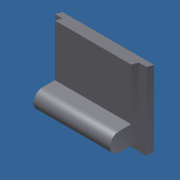
# Autodesk Inventor part: TETO DA CABINE(15)
Saved by Autodesk Inventor 2012 SP1 (Build 160190100, 190)
## iProperties
Created: 2012-07-23
Part Number: TETO DA CABINE(15)
Material: Carbon Steel
Document SubType Name: Modeling
Designer: bruno.silveira
Mass: 587.039 g
Surface Area: 115.824 cm^2
Volume: 74.592 cm^3
Density: 7.87 g/cm^3
Author: bruno.silveira
Autodesk Inventor part; units mm, degrees
ref_plane "YZ Plane" through (0, 0, 0) normal (1, 0, 0) x (0, 1, 0)
ref_plane "XZ Plane" through (0, 0, 0) normal (0, 1, 0) x (-1, 0, 0)
ref_plane "XY Plane" through (0, 0, 0) normal (0, 0, 1) x (1, 0, 0)
sketch "Sketch1" plane through (0, 0, 0) normal (0, 0, 1) x (1, 0, 0)
  line L0 (0, 0) -> (60, 0)
  line L1 (60, 0) -> (60, 24)
  line L2 (60, 24) -> (0, 24)
  line L3 (0, 24) -> (0, 0)
  dimension "d0" = 60
  dimension "d1" = 24
  constraints: 8 end point, 2 parallel, 1 horizontal, 1 perpendicular
  measures "d0" distance of L0.start L0.end
  measures "d1" distance of L2.end L0.start
extrude "Extrusion1" add sketch "Sketch1" along normal blind 51.8
sketch "Sketch2" plane through (60, 0, 0) normal (1, 0, 0) x (0, 0, -1)
  line L0 (-51.8, 24) -> (-51.8, 0) projected
  line L1 (0, 0) -> (-51.8, 0) projected
  line L2 (0, 0) -> (0, 24) projected
  line L3 (0, 24) -> (-51.8, 24) projected
  line L4 (-51.8, 14) -> (-18, 14)
  arc A0 (-18, 6) -> (-6, 6) centre (-12, 6) ccw
  line L5 (-18, 6) -> (-18, 14)
  line L6 (-6, 6) -> (-6, 19)
  line L7 (-6, 19) -> (0, 19)
  dimension "d5" = 10
  dimension "d6" = 18
  dimension "d7" = 12
  dimension "d8" = 5
  dimension "d9" = 6
  constraints: 8 end point, 2 parallel, 2 perpendicular, 2 point on circle, 2 point on line, 2 tangent, 1 centre point, 1 coincident
  measures "d5" distance between parallel lines of L3 L4
  measures "d6" distance from line of L3 point (-12, 6)
  measures "d7" diameter of A0
  measures "d8" distance from line of L3 L6.end
  measures "d9" distance between parallel lines of L2 L6
extrude "Extrusion2" cut sketch "Sketch2" against normal blind 60 contours L4 L5 A0 L1 L0 | L2 L1 A0 L6 L7
sketch "Sketch3" plane through (0, 0, 51.8) normal (0, 0, 1) x (1, 0, 0)
  line L0 (60, 0) -> (0, 0) projected
  line L1 (55, 19) -> (55, 0)
  line L2 (55, 0) -> (60, 0)
  line L3 (60, 0) -> (60, 19)
  line L4 (5, 19) -> (5, 0)
  line L5 (5, 0) -> (0, 0)
  line L6 (0, 0) -> (0, 19)
  line L7 (60, 19) -> (0, 19) projected
  line L8 (0, 24) -> (60, 24) projected
  line L9 (0, 0) -> (0, 24) projected
  line L10 (60, 24) -> (60, 0) projected
  line L11 (0, 19) -> (5, 19)
  line L12 (55, 19) -> (60, 19)
  point P0 (0, 14)
  point P1 (60, 14)
  dimension "d16" = 5
  dimension "d17" = 5
  constraints: 16 end point, 6 point on line, 2 collinear, 2 parallel
  measures "d16" distance of L1.start L3.end
  measures "d17" distance between parallel lines of L6 L4
extrude "Extrusion3" cut sketch "Sketch3" against normal blind 52 contours L0 L1 L7 L3 | L0 L6 L7 L4
chamfer "Chamfer1" distance 10 angle 15 1 edges at (30, 24, 51.8) measured on face at (21.6667, 22.3333, 51.8)
sketch "Sketch5" plane through (55, 19, 6) normal (0, 0, -1) x (-1, 0, 0)
  line L0 (0, 0) -> (0, -13) projected
  line L1 (-5, 5) -> (55, 5) projected
  point P0 (55, -19)
  point P1 (6, -9)
  point P2 (44, -9)
  dimension "d35" = 38
  dimension "d36" = 6
  dimension "d37" = 14
  dimension "d38" = 14
  measures "d35" distance of point (6, -9) point (44, -9)
  measures "d36" distance from line of L0 point (6, -9)
  measures "d37" distance from line of L1 point (6, -9)
  measures "d38" distance from line of L1 point (44, -9)
hole "Hole2" at (49, 10, 6) at (11, 10, 6) direction (0, 0, 1) diameter 4.917 depth 10 tip angle 118 thread size "M6x1" class "6H" standard "ANSI Metric M Profile"
chamfer "Chamfer2" distance 0.5 angle 45 2 edges at (11, 7.5415, 6) (49, 7.5415, 6)
body "Solid1"
